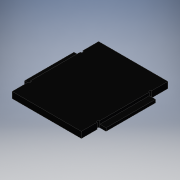
# Autodesk Inventor part: コックピット_2_サブフレーム_1
Saved by Autodesk Inventor 2018 (Build 220112000, 112)
## iProperties
Created: 2016-05-24
Part Number: コックピット_2_サブフレーム_1
Material: アセタール樹脂、黒
Document SubType Name: Modeling
Designer: hiroaki
Density: 1.425 g/cm^3
Appearance: 滑らか - 黒
Mass: 14.5273 g
Surface Area: 66.6596 cm^2
Volume: 10.1946 cm^3
Author: hiroaki
Autodesk Inventor part; units mm, degrees
ref_plane "YZ Plane" through (0, 0, 0) normal (1, 0, 0) x (0, 1, 0)
ref_plane "XZ Plane" through (0, 0, 0) normal (0, 1, 0) x (-1, 0, 0)
ref_plane "XY Plane" through (0, 0, 0) normal (0, 0, 1) x (1, 0, 0)
sketch "スケッチ1" plane through (0, 0, 0) normal (0, 0, 1) x (1, 0, 0)
  line L0 (-28, -35) -> (28, -35) construction
  line L1 (28, -35) -> (28, 35) construction
  line L2 (28, 35) -> (-28, 35) construction
  line L3 (-28, 35) -> (-28, -35) construction
  line L4 (-28, -35) -> (28, 35) construction
  line L5 (28, -35) -> (-28, 35) construction
  line L6 (-28, 22.1) -> (-28, 35)
  line L7 (-28, 35) -> (28, 35)
  line L8 (28, 35) -> (28, 22.1)
  line L9 (-28, 20) -> (-33, 20)
  line L10 (-33, 20) -> (-33, -20)
  line L11 (-33, -20) -> (-28, -20)
  line L12 (-28, -22.1) -> (-28, -35)
  line L13 (-28, -35) -> (28, -35)
  line L14 (28, -35) -> (28, -22.1)
  line L15 (28, 20) -> (33, 20)
  line L16 (33, 20) -> (33, -20)
  line L17 (33, -20) -> (28, -20)
  arc A0 (-28, 20) -> (-28, 22.1) centre (-28, 21.05) ccw
  arc A1 (-28, -22.1) -> (-28, -20) centre (-28, -21.05) ccw
  arc A2 (28, -20) -> (28, -22.1) centre (28, -21.05) ccw
  line L18 (0, 0) -> (0, 35) construction
  line L19 (0, 0) -> (28, 0) construction
  arc A3 (28, 22.1) -> (28, 20) centre (28, 21.05) ccw
  dimension "d9" = 56
  dimension "d12" = 70
  dimension "d13" = 15
  dimension "d39" = 15
  dimension "d40" = 1.05
  dimension "d41" = 5
  constraints: 40 end point, 10 perpendicular, 8 point on circle, 5 symmetric about line, 4 centre point, 4 collinear, 4 midpoint, 4 point on line, 3 horizontal, 2 horizontal alignment, 2 parallel, 2 vertical, 1 equal radius, 1 tangent, 1 other
  measures "d9" distance of L1.end L2.end
  measures "d12" distance of L0.end L1.end
  measures "d13" distance between parallel lines of L9 L2
  measures "d39" distance between parallel lines of L0 L11
  measures "d40" radius of A0
  measures "d41" distance of L9.start L9.end
extrude "押し出し1" add sketch "スケッチ1" along normal blind 5
sketch "スケッチ2" plane through (0, 0, 5) normal (0, 0, 1) x (1, 0, 0)
  line L0 (-28, 35) -> (-28, 22.1) projected
  line L1 (28, 35) -> (-28, 35) projected
  line L2 (-67.7785, 43.014) -> (-28, 43.014)
  line L3 (-28, 43.014) -> (-28, -43.014)
  line L4 (-28, -43.014) -> (-67.7785, -43.014)
  line L5 (-67.7785, -43.014) -> (-67.7785, 43.014)
  line L6 (67.7785, 43.014) -> (28, 43.014)
  line L7 (28, 43.014) -> (28, -43.014)
  line L8 (28, -43.014) -> (67.7785, -43.014)
  line L9 (67.7785, -43.014) -> (67.7785, 43.014)
  line L10 (0, 0) -> (0, 35) construction
  line L11 (0, 0) -> (33, 0) construction
  line L12 (33, 20) -> (33, -20) construction
  constraints: 20 end point, 4 parallel, 2 horizontal, 2 midpoint, 2 perpendicular, 2 symmetric about line, 1 collinear, 3 other
extrude "押し出し2" cut sketch "スケッチ2" against normal blind 2.5
equation "\"d12\" = d18"
equation "\"d13\" = d28"
equation "\"d39\" = d13"
equation "\"d18\" = 70"
equation "\"d28\" = 15"
